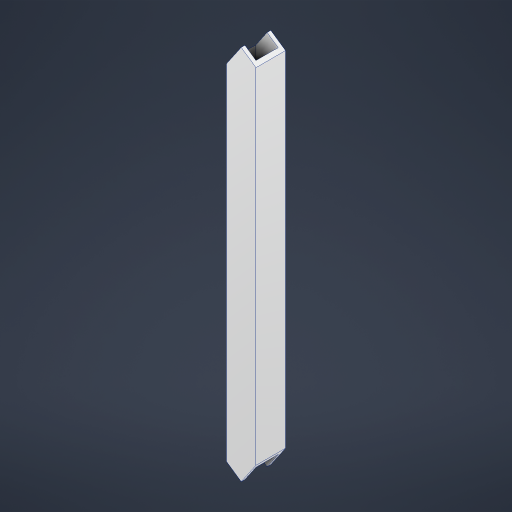
# Autodesk Inventor part: STRU_014_BilletCrossbar3_Angled
Saved by Autodesk Inventor 2024.2 (Build 282272000, 272)
## iProperties
Created: 2024-07-25
Part Number: STRU_014_BilletCrossbar3_Angled
Material: Aluminum 6061
Document SubType Name: Modeling
Designer: Bryan
Density: 2.7 g/cm^3
Appearance: Aluminum - Flat
Author: Bryan
Autodesk Inventor part; units mm, degrees
ref_plane "YZ Plane" through (0, 0, 0) normal (1, 0, 0) x (0, 1, 0)
ref_plane "XZ Plane" through (0, 0, 0) normal (0, 1, 0) x (-1, 0, 0)
ref_plane "XY Plane" through (0, 0, 0) normal (0, 0, 1) x (1, 0, 0)
sketch "Sketch1" plane through (0, 0, 0) normal (0, 1, 0) x (-1, 0, 0)
  line L0 (-12.7, -12.7) -> (12.7, -12.7)
  line L1 (12.7, -12.7) -> (12.7, 12.7)
  line L2 (12.7, 12.7) -> (-12.7, 12.7)
  line L3 (-12.7, 12.7) -> (-12.7, -12.7)
  line L4 (-12.7, -12.7) -> (12.7, 12.7) construction
  line L5 (12.7, -12.7) -> (-12.7, 12.7) construction
  line L6 (9.525, 9.525) -> (9.525, -9.525)
  line L7 (9.525, -9.525) -> (-9.525, -9.525)
  line L8 (-9.525, -9.525) -> (-9.525, 9.525)
  line L9 (-9.525, 9.525) -> (9.525, 9.525)
  point P0 (0, 0)
  dimension "d0" = 25.4
  dimension "d1" = 25.4
  dimension "d2" = 3.175
  constraints: 20 end point, 4 parallel, 2 midpoint, 2 perpendicular, 1 horizontal, 3 other
  measures "d0" distance of L2.end L1.end
  measures "d1" distance of L1.end L0.end
  measures "d2" distance between parallel lines of L1 L6
extrude "Extrusion1" add sketch "Sketch1" along normal blind 323.3735
sketch "Sketch2" plane through (-12.7, 0, 12.7) normal (0, 0, 1) x (1, 0, 0)
  line L0 (0, 0) -> (25.4, 0) projected
  line L1 (25.4, 0) -> (25.4, 323.3735) projected
  line L2 (0, 323.3735) -> (25.4, 323.3735) projected
  line L3 (0, 0) -> (0, 323.3735) projected
  line L4 (163.521, 219.9589) -> (12.7, 323.3735)
  line L5 (12.7, 323.3735) -> (-138.121, 103.4146)
  line L6 (-138.121, 103.4146) -> (12.7, 0)
  line L7 (12.7, 0) -> (163.521, 219.9589)
  point P0 (0, 8.7081)
  point P1 (25.4, 18.5218)
  point P2 (0, 304.8517)
  point P3 (25.4, 314.6654)
  dimension "d5" = 266.7
  constraints: 8 end point, 2 midpoint, 2 parallel, 1 perpendicular
  measures "d5" distance of L4.end L5.end
extrude "Extrusion2" cut sketch "Sketch2" against normal through all contours L3 L6 L0 | L7 L1 L0 | L3 L2 L5 | L4 L2 L1
body "Solid1"
